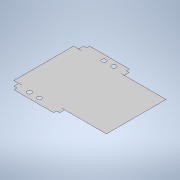
# Autodesk Inventor part: Slab Template- 1 piece v1
Saved by Autodesk Inventor 2022 (Build 260153000, 153)
## iProperties
Created: 2021-09-30
Part Number: Slab Template- 1 piece v1
Material: Generic
Document SubType Name: Modeling
Designer: Administrator
Density: 1 g/cm^3
Appearance: Default
Title: Slab Template- 1 piece v1 v1
Author: Administrator
Autodesk Inventor part; units mm, degrees
ref_plane "YZ Plane" through (0, 0, 0) normal (1, 0, 0) x (0, 1, 0)
ref_plane "XZ Plane" through (0, 0, 0) normal (0, 1, 0) x (-1, 0, 0)
ref_plane "XY Plane" through (0, 0, 0) normal (0, 0, 1) x (1, 0, 0)
sketch "Sketch1" plane through (0, 0, 0) normal (0, 1, 0) x (-1, 0, 0)
  line L0 (-465, -380) -> (465, -380)
  line L1 (465, -380) -> (465, 380)
  line L2 (465, 380) -> (-465, 380)
  line L3 (-465, 380) -> (-465, -380)
  line L4 (-465, -380) -> (465, 380) construction
  line L5 (465, -380) -> (-465, 380) construction
  point P0 (0, 0)
  dimension "d0" = 930
  dimension "d1" = 760
  constraints: 12 end point, 2 midpoint, 2 parallel, 1 horizontal, 1 perpendicular
  measures "d0" distance of L1.end L2.end
  measures "d1" distance of L0.end L1.end
extrude "Extrusion1" add sketch "Sketch1" along normal blind 0.1
sketch "Sketch5" plane through (0, 0.1, 0) normal (0, 1, 0) x (1, 0, 0)
  line L0 (-465, -380) -> (465, -380) projected
  line L1 (465, -380) -> (65, -380)
  line L2 (65, -380) -> (65, -300)
  line L3 (65, -300) -> (465, -300)
  line L4 (465, -300) -> (465, -380)
  line L5 (465, -380) -> (465, 380) projected
  line L6 (465, 380) -> (65, 380)
  line L7 (65, 380) -> (65, 300)
  line L8 (65, 300) -> (465, 300)
  line L9 (465, 300) -> (465, 380)
  line L10 (-465, 380) -> (-465, -380) projected
  line L11 (-465, -380) -> (-435, -380)
  line L12 (-435, -380) -> (-435, -300)
  line L13 (-435, -300) -> (-465, -300)
  line L14 (-465, -300) -> (-465, -380)
  line L15 (-465, 380) -> (-435, 380)
  line L16 (-435, 380) -> (-435, 300)
  line L17 (-435, 300) -> (-465, 300)
  line L18 (-465, 300) -> (-465, 380)
  point P0 (0, 0)
  point P1 (65, -380)
  dimension "d33" = 80
  dimension "d34" = 80
  dimension "d35" = 400
  dimension "d36" = 400
  dimension "d37" = 80
  dimension "d38" = 80
  dimension "d39" = 30
  constraints: 32 end point, 8 parallel, 4 horizontal, 4 perpendicular, 1 point on line
  measures "d33" distance of L1.end L2.end
  measures "d34" distance of L6.end L7.end
  measures "d35" distance of L2.end L3.end
  measures "d36" distance of L7.end L8.end
  measures "d37" distance of L11.end L12.end
  measures "d38" distance of L15.end L16.end
  measures "d39" distance of L12.end L13.end
extrude "Extrusion4" cut sketch "Sketch5" against normal through all
sketch "Sketch6" plane through (0, 0.1, 0) normal (0, 1, 0) x (1, 0, 0)
  line L0 (-435, -380) -> (65, -380) projected
  line L1 (-435, -380) -> (-415, -380)
  line L2 (-415, -380) -> (-415, -300)
  line L3 (-415, -300) -> (-435, -300)
  line L4 (-435, -300) -> (-435, -380)
  line L5 (-415, -380) -> (-385, -380)
  line L6 (-385, -380) -> (-385, -350)
  line L7 (-385, -350) -> (-415, -350)
  line L8 (-415, -350) -> (-415, -380)
  line L9 (65, -300) -> (65, -380) projected
  line L10 (65, -380) -> (45, -380)
  line L11 (45, -380) -> (45, -300)
  line L12 (45, -300) -> (65, -300)
  line L13 (65, -300) -> (65, -380)
  line L14 (45, -380) -> (15, -380)
  line L15 (15, -380) -> (15, -350)
  line L16 (15, -350) -> (45, -350)
  line L17 (45, -350) -> (45, -380)
  line L18 (65, 300) -> (65, 380) projected
  line L19 (65, 380) -> (45, 380)
  line L20 (45, 380) -> (45, 300)
  line L21 (45, 300) -> (65, 300)
  line L22 (65, 300) -> (65, 380)
  line L23 (45, 380) -> (15, 380)
  line L24 (15, 380) -> (15, 350)
  line L25 (15, 350) -> (45, 350)
  line L26 (45, 350) -> (45, 380)
  line L27 (65, 380) -> (-435, 380) projected
  line L28 (-435, 380) -> (-415, 380)
  line L29 (-415, 380) -> (-415, 300)
  line L30 (-415, 300) -> (-435, 300)
  line L31 (-435, 300) -> (-435, 380)
  line L32 (-415, 380) -> (-385, 380)
  line L33 (-385, 380) -> (-385, 350)
  line L34 (-385, 350) -> (-415, 350)
  line L35 (-415, 350) -> (-415, 380)
  point P0 (0, 0)
  dimension "d42" = 30
  dimension "d43" = 30
  dimension "d44" = 80
  dimension "d45" = 20
  dimension "d46" = 30
  dimension "d47" = 30
  dimension "d48" = 20
  dimension "d49" = 20
  dimension "d50" = 30
  dimension "d51" = 30
  dimension "d52" = 80
  dimension "d53" = 20
  dimension "d54" = 30
  dimension "d55" = 30
  constraints: 64 end point, 16 parallel, 8 horizontal, 8 perpendicular, 2 point on line
  measures "d42" distance of L6.end L7.end
  measures "d43" distance of L5.end L6.end
  measures "d44" distance of L1.end L2.end
  measures "d45" distance of L2.end L3.end
  measures "d46" distance of L14.end L15.end
  measures "d47" distance of L15.end L16.end
  measures "d48" distance of L11.end L12.end
  measures "d49" distance of L20.end L21.end
  measures "d50" distance of L23.end L24.end
  measures "d51" distance of L24.end L25.end
  measures "d52" distance of L21.end L18.end
  measures "d53" distance of L29.end L30.end
  measures "d54" distance of L33.end L34.end
  measures "d55" distance of L32.end L33.end
extrude "Extrusion5" cut sketch "Sketch6" against normal through all
sketch "Sketch7" plane through (0, 0.1, 0) normal (0, 1, 0) x (1, 0, 0)
  circle A0 centre (-285, -325) radius 22.5
  circle A1 centre (-185, -325) radius 22.5
  line L0 (-415, -350) -> (-385, -350) projected
  line L1 (-385, -350) -> (-385, -380) projected
  circle A2 centre (-85, 325) radius 22.5
  circle A3 centre (-185, 325) radius 22.5
  line L2 (45, 350) -> (15, 350) projected
  line L3 (15, 350) -> (15, 380) projected
  point P0 (0, 0)
  dimension "d58" = 45
  dimension "d59" = 45
  dimension "d60" = 25
  dimension "d61" = 100
  dimension "d62" = 200
  dimension "d63" = 45
  dimension "d64" = 45
  dimension "d65" = 25
  dimension "d66" = 100
  dimension "d67" = 200
  constraints: 4 centre point, 2 horizontal alignment
  measures "d58" diameter of A0
  measures "d59" diameter of A1
  measures "d60" distance from line of L0 A0.centre
  measures "d61" distance from line of L1 A0.centre
  measures "d62" distance from line of A1.centre L1
  measures "d63" diameter of A2
  measures "d64" diameter of A3
  measures "d65" distance from line of A2.centre L2
  measures "d66" distance from line of A2.centre L3
  measures "d67" distance from line of A3.centre L3
extrude "Extrusion6" cut sketch "Sketch7" against normal through all
sketch "Sketch8" plane through (0, 0.1, 0) normal (0, 1, 0) x (1, 0, 0)
  line L0 (-415, -300) -> (-465, -300) projected
  line L1 (-415, -300) -> (-385, -300)
  line L2 (-385, -300) -> (-385, -300.2)
  line L3 (-385, -300.2) -> (-415, -300.2)
  line L4 (-415, -300.2) -> (-415, -300)
  line L5 (-415, 300) -> (-415, 350) projected
  line L6 (-415, 300) -> (-385, 300)
  line L7 (-385, 300) -> (-385, 300.2)
  line L8 (-385, 300.2) -> (-415, 300.2)
  line L9 (-415, 300.2) -> (-415, 300)
  line L10 (45, -300) -> (45, -350) projected
  line L11 (45, -300) -> (15, -300)
  line L12 (15, -300) -> (15, -300.2)
  line L13 (15, -300.2) -> (45, -300.2)
  line L14 (45, -300.2) -> (45, -300)
  line L15 (45, 300) -> (45, 350) projected
  line L16 (45, 300) -> (15, 300)
  line L17 (15, 300) -> (15, 300.2)
  line L18 (15, 300.2) -> (45, 300.2)
  line L19 (45, 300.2) -> (45, 300)
  point P0 (0, 0)
  dimension "d70" = 30
  dimension "d72" = 0.2
  dimension "d74" = 30
  dimension "d75" = 0.2
  dimension "d76" = 0.2
  dimension "d77" = 30
  dimension "d78" = 0.2
  dimension "d79" = 30
  constraints: 32 end point, 8 parallel, 4 horizontal, 4 perpendicular
  measures "d70" distance of L2.end L3.end
  measures "d72" distance of L1.end L2.end
  measures "d74" distance of L7.end L8.end
  measures "d75" distance of L6.end L7.end
  measures "d76" distance of L11.end L12.end
  measures "d77" distance of L12.end L13.end
  measures "d78" distance of L16.end L17.end
  measures "d79" distance of L17.end L18.end
extrude "Extrusion7" cut sketch "Sketch8" against normal through all
equation "\"d34\" = d33"
equation "\"d36\" = d35"
equation "\"d37\" = d33"
equation "\"d38\" = d33"
equation "\"d46\" = d43"
equation "\"d47\" = d42"
equation "\"d48\" = d45"
equation "\"d49\" = d45"
equation "\"d50\" = d43"
equation "\"d51\" = d42"
equation "\"d52\" = d44"
equation "\"d53\" = d45"
equation "\"d54\" = d42"
equation "\"d55\" = d43"
equation "\"d59\" = d58"
equation "\"d63\" = d59"
equation "\"d64\" = d58"
equation "\"d65\" = d60"
equation "\"d66\" = d61"
equation "\"d67\" = d62"
equation "\"d74\" = d70"
equation "\"d75\" = d72"
equation "\"d76\" = d72"
equation "\"d77\" = d70"
equation "\"d78\" = d72"
equation "\"d79\" = d70"
body "Solid2"
